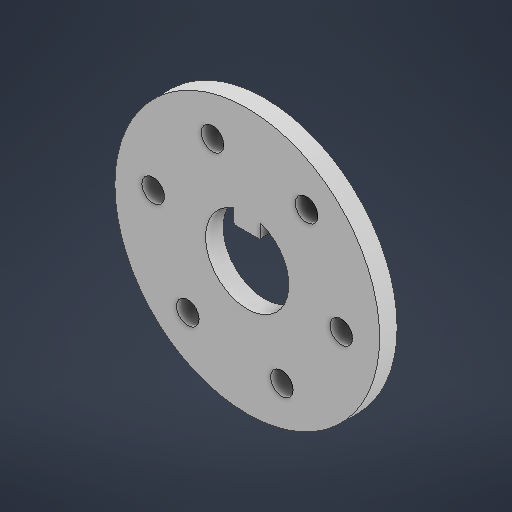
# Autodesk Inventor part: spool_spacer_driver
Saved by Autodesk Inventor 2026.1 (Build 301233000, 233)
## iProperties
Created: 2026-04-28
Part Number: spool_spacer_driver
Material: Generic
Document SubType Name: Modeling
Designer: aaron
Density: 1 g/cm^3
Appearance: Default
Author: aaron
Autodesk Inventor part; units mm, degrees
ref_plane "YZ Plane" through (0, 0, 0) normal (1, 0, 0) x (0, 1, 0)
ref_plane "XZ Plane" through (0, 0, 0) normal (0, 1, 0) x (-1, 0, 0)
ref_plane "XY Plane" through (0, 0, 0) normal (0, 0, 1) x (1, 0, 0)
sketch "Sketch1" plane through (0, 0, 0) normal (0, 0, 1) x (1, 0, 0)
  circle A0 centre (0, 0) radius 24
  circle A1 centre (0, 0) radius 7.55
  dimension "d0" = 48
  dimension "d1" = 15.1
  constraints: 2 centre point, 2 coincident
  measures "d0" diameter of A0
  measures "d1" diameter of A1
extrude "Extrusion1" add sketch "Sketch1" along normal blind 3.18
sketch "Sketch2" plane through (0, 0, 0) normal (0, 0, -1) x (-1, 0, 0)
  circle A0 centre (-16.5319, -11.256) radius 2.05 projected
  circle A1 centre (-19.649, 3.7306) radius 2.05 projected
  circle A2 centre (-17.0544, -2.5903) radius 1.65 projected
  circle A3 centre (-6.284, -16.0647) radius 1.65 projected
  circle A4 centre (-6.284, -16.0647) radius 1.65
  circle A5 centre (-6.284, -16.0647) radius 2.125
  circle A6 centre (10.7704, -13.4744) radius 2.125
  circle A7 centre (17.0544, 2.5903) radius 2.125
  circle A8 centre (6.284, 16.0647) radius 2.125
  circle A9 centre (-10.7704, 13.4744) radius 2.125
  circle A10 centre (-17.0544, -2.5903) radius 2.125
  point P0 (0, 0)
  dimension "d4" = 4.25
  dimension "d7" = 360
  constraints: 7 centre point, 2 coincident, 1 concentric, 13 other
  measures "d4" diameter of A5
extrude "Extrusion2" cut sketch "Sketch2" against normal through all contours A2 | A3 | A5 | A6 | A7 | A8 | A9 | A10
sketch "Sketch3" plane through (0, 0, 3.18) normal (0, 0, 1) x (1, 0, 0)
  line L0 (-2.5, 4.5) -> (-2.5, 7.0711)
  arc A0 (-2.5, 7.0711) -> (2.5, 7.0711) centre (0, 0) ccw
  line L1 (2.5, 7.0711) -> (2.5, 4.5)
  line L2 (2.5, 4.5) -> (-2.5, 4.5)
  line L3 (-2.4503, 4.5542) -> (2.4493, 4.5542)
  line L4 (2.4493, 4.5542) -> (2.4493, 8.0911)
  line L5 (2.4493, 8.0911) -> (-2.4503, 8.0911)
  line L6 (-2.4503, 8.0911) -> (-2.4503, 4.5542)
  circle A1 centre (0, 0) radius 7.55 projected
  dimension "d16" = 7.5
  dimension "d17" = 5
  dimension "d18" = 2.9958
  constraints: 14 end point, 2 parallel, 2 point on circle, 1 centre point, 1 horizontal, 1 perpendicular
  measures "d16" radius of A0
  measures "d17" distance between parallel lines of L1 L0
  measures "d18" distance edge to line of A1 L3
extrude "Extrusion3" add sketch "Sketch3" against normal up to surface (3.18 mm away) contours L6 A1 L4 L3 | L6 L5 L4 A1 picked at (-0.2772, 5.5375)
chamfer "Chamfer1" distance 0.2 angle 45 2 edges at (-2.4503, 4.5542, 1.59) (2.4493, 4.5542, 1.59)
sketch "Sketch4" plane through (0, 0, 3.18) normal (0, 0, 1) x (1, 0, 0)
  circle A0 centre (-6.284, 16.0647) radius 2.125 projected
  circle A1 centre (-6.284, 16.0647) radius 2.05
  line L0 (2.4493, 4.7542) -> (2.2493, 4.5542) projected
  line L1 (2.4493, 4.7542) -> (2.4493, 7.1417) projected
  arc A2 (-2.4503, 7.1413) -> (2.4493, 7.1417) centre (0, 0) ccw projected
  line L2 (-2.4503, 7.1413) -> (-2.4503, 4.7542) projected
  line L3 (-2.2503, 4.5542) -> (-2.4503, 4.7542) projected
  line L4 (-2.2503, 4.5542) -> (2.2493, 4.5542) projected
  circle A3 centre (-17.0544, 2.5903) radius 2.125 projected
  circle A4 centre (6.284, -16.0647) radius 2.125 projected
  circle A5 centre (-10.7704, -13.4744) radius 2.125 projected
  circle A6 centre (-6.284, 16.0647) radius 2.125 projected
  circle A7 centre (17.0544, -2.5903) radius 2.125 projected
  circle A8 centre (10.7704, 13.4744) radius 2.125 projected
  circle A9 centre (0, 0) radius 24 projected
  circle A10 centre (-17.0544, 2.5903) radius 2.05
  circle A11 centre (-10.7704, -13.4744) radius 2.05
  circle A12 centre (6.284, -16.0647) radius 2.05
  circle A13 centre (17.0544, -2.5903) radius 2.05
  circle A14 centre (10.7704, 13.4744) radius 2.05
  dimension "d19" = 4.1
  dimension "d22" = 360
  constraints: 6 centre point, 1 coincident, 13 other
  measures "d19" diameter of A1
extrude "Extrusion4" add sketch "Sketch4" against normal up to surface (3.18 mm away) contours A0 | A3 | A4 | A5 | A7 | A8
body "Solid1"
